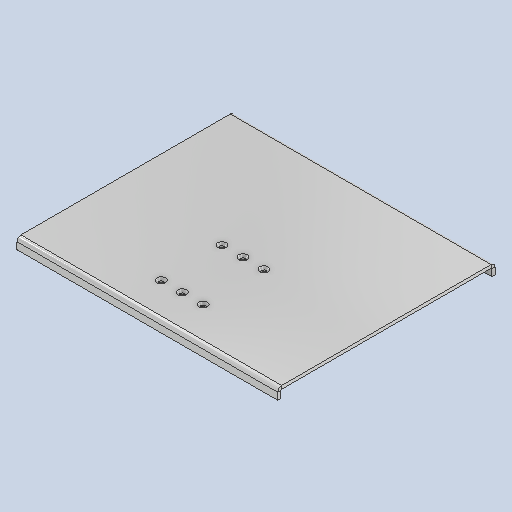
# Autodesk Inventor part: axis_12_bottom_frame(bottom)
Saved by Autodesk Inventor 2025.2 (Build 292293000, 293)
## iProperties
Created: 2025-05-04
Part Number: axis_12_bottom_frame(bottom)
Material: Aluminum 6061-AHC
Document SubType Name: Sheet Metal
Designer: User
Density: 2.7 g/cm^3
Sheet Metal Rule: Default_mm
Appearance: Aluminum - Dark
Author: User
Autodesk Inventor part; units mm, degrees
ref_plane "YZ Plane" through (0, 0, 0) normal (1, 0, 0) x (0, 1, 0)
ref_plane "XZ Plane" through (0, 0, 0) normal (0, 1, 0) x (-1, 0, 0)
ref_plane "XY Plane" through (0, 0, 0) normal (0, 0, 1) x (1, 0, 0)
sketch "Sketch1" plane through (0, 0, 0) normal (0, 1, 0) x (-1, 0, 0)
  line L0 (60, -50) -> (-60, -50)
  line L1 (-60, -50) -> (-60, 50)
  line L2 (-60, 50) -> (60, 50)
  line L3 (60, 50) -> (60, -50)
  point P0 (0, 0)
  dimension "d0" = 120
  dimension "d1" = 100
  dimension "d2" = 50
  dimension "d3" = 60
  measures "d0" distance of L0.start L0.end
  measures "d1" distance of L0.end L1.end
  measures "d2" distance from line of L0 point (0, 0)
  measures "d3" distance from line of point (0, 0) L3
extrude "Plate1" add sketch "Sketch1" along normal blind 1.5
sketch "Sketch2" plane through (60, 1.5, -48.5) normal (0, 0, -1) x (-1, 0, 0)
  line L0 (120, 0) -> (0, 0)
  line L1 (0, 0) -> (0, -5)
  line L2 (0, -5) -> (120, -5)
  line L3 (120, -5) -> (120, 0)
  constraints: 6 end point, 1 horizontal, 1 perpendicular, 1 vertical
edge flange "Flange1" height 5 angle 90 thickness 1.5 bend radius 0.31 thickness toward (0, 0, -1) relief straight relief width 1.5 relief depth 0.75 corner gap 0.31 corner form 0 edges at (0, 0, -50) (0, 0, 50) wall of the first edge with corners at (-60, 1.5, -48.5) (60, 1.5, -48.5) (60, -3.5, -48.5) (-60, -3.5, -48.5)
bend "Bend1"
corner "Corner1"
sketch "Sketch3" plane through (0, 1.5, 0) normal (0, 1, 0) x (1, 0, 0)
  circle A0 centre (9.655, -34) radius 1.05 projected
  circle A1 centre (9.655, -6) radius 1.05 projected
  circle A2 centre (0, -34) radius 1.05 projected
  circle A3 centre (0, -6) radius 1.05 projected
  circle A4 centre (-9.655, -34) radius 1.05 projected
  circle A5 centre (-9.655, -6) radius 1.05 projected
  line L0 (15.655, 0) -> (15.655, -40) projected
  line L1 (-15.655, -40) -> (15.655, -40) projected
  line L2 (-15.655, -40) -> (-15.655, 0) projected
  line L3 (15.655, 0) -> (-15.655, 0) projected
  point P0 (0, 0)
  constraints: 1 other
hole "Hole1" at (-9.655, 1.5, 6) at (0, 1.5, 6) at (9.655, 1.5, 6) at (9.655, 1.5, 34) at (0, 1.5, 34) at (-9.655, 1.5, 34) direction (0, -1, 0) diameter 2.1 depth 1.5 countersink diameter 4 countersink angle 90
equation "\"d20\" = Thickness"
equation "\"d4\" = Thickness"
equation "\"d5\" = BendReliefWidth"
equation "\"d6\" = BendReliefDepth"
equation "\"d7\" = MinimumRemnant"
equation "\"d8\" = TransitionRadius"
equation "\"d11\" = BendRadius"
equation "\"d12\" = CornerReliefSize"
equation "\"d13\" = GapSize"
equation "\"d14\" = JacobiRadiusSize"
equation "\"BendReliefWidth\" = Thickness"
equation "\"BendReliefDepth\" = 0.5 * Thickness"
equation "\"CornerReliefSize\" = 4 * Thickness"
equation "\"MinimumRemnant\" = 2 * Thickness"
equation "\"TransitionRadius\" = BendRadius"
equation "\"JacobiRadiusSize\" = BendRadius"
equation "\"GapSize\" = Thickness"
equation "\"Thickness\" = 1.5"
equation "\"BendRadius\" = 0.31"
body "Solid1"
